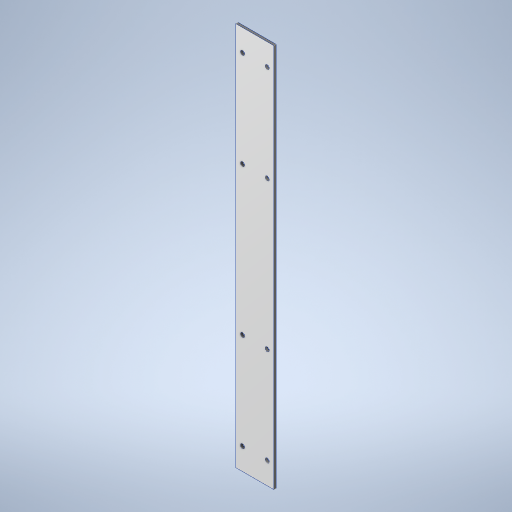
# Autodesk Inventor part: Narrow Internal Vertical Side Panels
Saved by Autodesk Inventor 2024 (Build 280153000, 153)
## iProperties
Created: 2024-09-28
Part Number: Narrow Internal Vertical Side Panels
Material: Generic
Document SubType Name: Modeling
Designer: Ishaan
Density: 1 g/cm^3
Appearance: Default
Author: Ishaan
Autodesk Inventor part; units mm, degrees
ref_plane "YZ Plane" through (0, 0, 0) normal (1, 0, 0) x (0, 1, 0)
ref_plane "XZ Plane" through (0, 0, 0) normal (0, 1, 0) x (-1, 0, 0)
ref_plane "XY Plane" through (0, 0, 0) normal (0, 0, 1) x (1, 0, 0)
sketch "Sketch1" plane through (0, 0, 0) normal (0, 0, 1) x (1, 0, 0)
  line L0 (24.75, -249.5) -> (-24.75, -249.5)
  line L1 (-24.75, -249.5) -> (-24.75, 249.5)
  line L2 (-24.75, 249.5) -> (24.75, 249.5)
  line L3 (24.75, 249.5) -> (24.75, -249.5)
  line L4 (24.75, -249.5) -> (-24.75, 249.5) construction
  line L5 (-24.75, -249.5) -> (24.75, 249.5) construction
  point P0 (0, 0)
  dimension "d0" = 49.5
  dimension "d1" = 499
  constraints: 12 end point, 2 midpoint, 2 parallel, 1 horizontal, 1 perpendicular
  measures "d0" distance of L1.end L2.end
  measures "d1" distance of L0.end L1.end
extrude "Extrusion1" add sketch "Sketch1" along normal mid plane 3
extrude "Extrusion2" cut sketch "Sketch1" along normal mid plane 2.9
extrude "Extrusion3" add sketch "Sketch1" along normal mid plane 2.9 separate body
sketch "Sketch2" plane through (0, 0, 1.5) normal (0, 0, 1) x (1, 0, 0)
  line L0 (16, -221) -> (-16, -221)
  line L1 (-16, -221) -> (-16, 221)
  line L2 (-16, 221) -> (16, 221)
  line L3 (16, 221) -> (16, -221)
  line L4 (16, -221) -> (-16, 221) construction
  line L5 (-16, -221) -> (16, 221) construction
  line L6 (16, -96) -> (-16, -96)
  line L7 (-16, -96) -> (-16, 96)
  line L8 (-16, 96) -> (16, 96)
  line L9 (16, 96) -> (16, -96)
  line L10 (16, -96) -> (-16, 96) construction
  line L11 (-16, -96) -> (16, 96) construction
  line L12 (-24.75, -249.5) -> (24.75, -249.5) projected
  point P0 (0, 0)
  dimension "d8" = 32
  dimension "d10" = 442
  dimension "d11" = 125
  constraints: 24 end point, 8 coincident, 4 midpoint, 4 parallel, 2 horizontal, 2 perpendicular, 1 point on line
  measures "d8" distance of L1.end L2.end
  measures "d10" distance of L2.end L0.start
  measures "d11" distance between parallel lines of L0 L6
hole "Hole1" at (-16, 221, 1.5) at (16, 221, 1.5) at (-16, 96, 1.5) at (16, 96, 1.5) at (-16, -96, 1.5) at (16, -96, 1.5) at (16, -221, 1.5) at (-16, -221, 1.5) direction (0, 0, -1) diameter 5.4 end through all bodies 1 2
